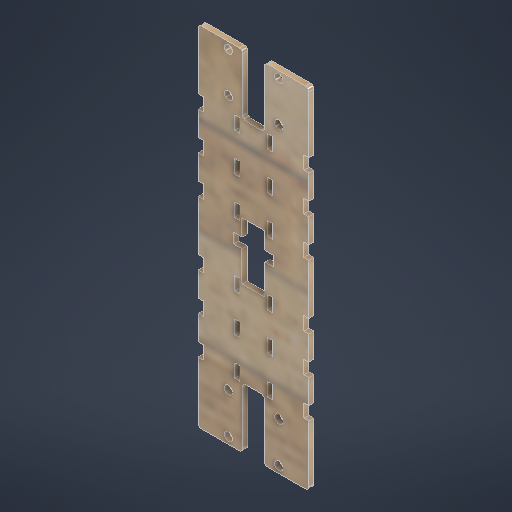
# Autodesk Inventor part: frame_v2
Saved by Autodesk Inventor 2025.3 (Build 293356030, 356C)
## iProperties
Created: 2025-09-03
Part Number: frame_v2
Material: 木材 (楓木)
Document SubType Name: Modeling
Designer: 陳泓任
Density: 0.67 g/cm^3
Appearance: 天然楓木 - 深色亮面處理
Author: 陳泓任
Autodesk Inventor part; units mm, degrees
ref_plane "YZ Plane" through (0, 0, 0) normal (1, 0, 0) x (0, 1, 0)
ref_plane "XZ Plane" through (0, 0, 0) normal (0, 1, 0) x (-1, 0, 0)
ref_plane "XY Plane" through (0, 0, 0) normal (0, 0, 1) x (1, 0, 0)
sketch "草圖1" plane through (0, 0, 0) normal (0, 0, 1) x (1, 0, 0)
  line L0 (-33, -104) -> (33, 104) construction
  line L1 (33, -104) -> (-33, 104) construction
  line L2 (0, 128.5379) -> (0, -160.5456)
  circle A0 centre (-15, 100) radius 2.5
  circle A1 centre (15, 100) radius 2.5
  circle A2 centre (15, 76) radius 2.5
  circle A3 centre (-15, 76) radius 2.5
  line L3 (-33, 68) -> (-30, 68)
  line L4 (-30, 68) -> (-30, 60)
  line L5 (-30, 60) -> (-33, 60)
  line L6 (-33, 102) -> (-33, 68)
  line L7 (-11.2, 68) -> (-8.2, 68)
  line L8 (-8.2, 68) -> (-8.2, 60)
  line L9 (-8.2, 60) -> (-11.2, 60)
  line L10 (-11.2, 60) -> (-11.2, 68)
  line L11 (33, 68) -> (30, 68)
  line L12 (30, 68) -> (30, 60)
  line L13 (30, 60) -> (33, 60)
  line L14 (11.2, 68) -> (8.2, 68)
  line L15 (8.2, 68) -> (8.2, 60)
  line L16 (8.2, 60) -> (11.2, 60)
  line L17 (11.2, 60) -> (11.2, 68)
  line L18 (33, 68) -> (33, 102)
  line L19 (8.2, 45.5) -> (8.2, 37.5)
  line L20 (8.2, 37.5) -> (11.2, 37.5)
  line L21 (11.2, 45.5) -> (8.2, 45.5)
  line L22 (11.2, 37.5) -> (11.2, 45.5)
  line L23 (30, 45.5) -> (30, 37.5)
  line L24 (30, 37.5) -> (33, 37.5)
  line L25 (33, 45.5) -> (30, 45.5)
  line L26 (-8.2, 45.5) -> (-8.2, 37.5)
  line L27 (-8.2, 37.5) -> (-11.2, 37.5)
  line L28 (-11.2, 45.5) -> (-8.2, 45.5)
  line L29 (-11.2, 37.5) -> (-11.2, 45.5)
  line L30 (-30, 45.5) -> (-30, 37.5)
  line L31 (-33, 45.5) -> (-30, 45.5)
  line L32 (-30, 37.5) -> (-33, 37.5)
  line L33 (8.2, 23) -> (8.2, 15)
  line L34 (8.2, 15) -> (11.2, 15)
  line L35 (11.2, 23) -> (8.2, 23)
  line L36 (11.2, 15) -> (11.2, 23)
  line L37 (30, 23) -> (30, 15)
  line L38 (30, 15) -> (33, 15)
  line L39 (33, 23) -> (30, 23)
  line L40 (-8.2, 23) -> (-8.2, 15)
  line L41 (-8.2, 15) -> (-11.2, 15)
  line L42 (-11.2, 23) -> (-8.2, 23)
  line L43 (-11.2, 15) -> (-11.2, 23)
  line L44 (-30, 23) -> (-30, 15)
  line L45 (-33, 23) -> (-30, 23)
  line L46 (-30, 15) -> (-33, 15)
  line L47 (-33, 60) -> (-33, 45.5)
  line L48 (-33, 37.5) -> (-33, 23)
  line L49 (33, 23) -> (33, 37.5)
  line L50 (33, 45.5) -> (33, 60)
  line L51 (-4.5, 68) -> (4.5, 68)
  line L52 (6.5, 70) -> (6.5, 102)
  line L53 (-6.5, 102) -> (-6.5, 70)
  line L54 (-6.5, 68) -> (6.5, 104) construction
  line L55 (6.5, 68) -> (-6.5, 104) construction
  line L56 (31, 104) -> (8.5, 104)
  line L57 (-8.5, 104) -> (-31, 104)
  arc A4 (-6.5, 102) -> (-8.5, 104) centre (-8.5, 102) ccw
  arc A5 (8.5, 104) -> (6.5, 102) centre (8.5, 102) ccw
  arc A6 (-6.5, 70) -> (-4.5, 68) centre (-4.5, 70) ccw
  arc A7 (4.5, 68) -> (6.5, 70) centre (4.5, 70) ccw
  arc A8 (-31, 104) -> (-33, 102) centre (-31, 102) ccw
  arc A9 (33, 102) -> (31, 104) centre (31, 102) ccw
  line L58 (-83.0249, 0) -> (86.2934, 0)
  circle A10 centre (-15, -100) radius 2.5
  circle A11 centre (15, -100) radius 2.5
  circle A12 centre (15, -76) radius 2.5
  circle A13 centre (-15, -76) radius 2.5
  line L59 (-33, -68) -> (-30, -68)
  line L60 (-30, -68) -> (-30, -60)
  line L61 (-30, -60) -> (-33, -60)
  line L62 (-33, -102) -> (-33, -68)
  line L63 (-11.2, -68) -> (-8.2, -68)
  line L64 (-8.2, -68) -> (-8.2, -60)
  line L65 (-8.2, -60) -> (-11.2, -60)
  line L66 (-11.2, -60) -> (-11.2, -68)
  line L67 (33, -68) -> (30, -68)
  line L68 (30, -68) -> (30, -60)
  line L69 (30, -60) -> (33, -60)
  line L70 (8.2, -60) -> (11.2, -60)
  line L71 (11.2, -60) -> (11.2, -68)
  line L72 (8.2, -68) -> (8.2, -60)
  line L73 (11.2, -68) -> (8.2, -68)
  line L74 (33, -68) -> (33, -102)
  line L75 (8.2, -45.5) -> (8.2, -37.5)
  line L76 (8.2, -37.5) -> (11.2, -37.5)
  line L77 (11.2, -45.5) -> (8.2, -45.5)
  line L78 (11.2, -37.5) -> (11.2, -45.5)
  line L79 (30, -45.5) -> (30, -37.5)
  line L80 (30, -37.5) -> (33, -37.5)
  line L81 (33, -45.5) -> (30, -45.5)
  line L82 (-8.2, -45.5) -> (-8.2, -37.5)
  line L83 (-8.2, -37.5) -> (-11.2, -37.5)
  line L84 (-11.2, -45.5) -> (-8.2, -45.5)
  line L85 (-11.2, -37.5) -> (-11.2, -45.5)
  line L86 (-30, -45.5) -> (-30, -37.5)
  line L87 (-33, -45.5) -> (-30, -45.5)
  line L88 (-30, -37.5) -> (-33, -37.5)
  line L89 (8.2, -23) -> (8.2, -15)
  line L90 (8.2, -15) -> (11.2, -15)
  line L91 (11.2, -23) -> (8.2, -23)
  line L92 (11.2, -15) -> (11.2, -23)
  line L93 (30, -23) -> (30, -15)
  line L94 (30, -15) -> (33, -15)
  line L95 (33, -23) -> (30, -23)
  line L96 (-8.2, -23) -> (-8.2, -15)
  line L97 (-8.2, -15) -> (-11.2, -15)
  line L98 (-11.2, -23) -> (-8.2, -23)
  line L99 (-11.2, -15) -> (-11.2, -23)
  line L100 (-30, -23) -> (-30, -15)
  line L101 (-33, -23) -> (-30, -23)
  line L102 (-30, -15) -> (-33, -15)
  line L103 (-33, -60) -> (-33, -45.5)
  line L104 (-33, -37.5) -> (-33, -23)
  line L105 (33, -23) -> (33, -37.5)
  line L106 (33, -45.5) -> (33, -60)
  line L107 (-4.5, -68) -> (4.5, -68)
  line L108 (6.5, -70) -> (6.5, -102)
  line L109 (-6.5, -102) -> (-6.5, -70)
  line L110 (-6.5, -68) -> (6.5, -104) construction
  line L111 (6.5, -68) -> (-6.5, -104) construction
  line L112 (31, -104) -> (8.5, -104)
  line L113 (-8.5, -104) -> (-31, -104)
  arc A14 (-8.5, -104) -> (-6.5, -102) centre (-8.5, -102) ccw
  arc A15 (6.5, -102) -> (8.5, -104) centre (8.5, -102) ccw
  arc A16 (-4.5, -68) -> (-6.5, -70) centre (-4.5, -70) ccw
  arc A17 (6.5, -70) -> (4.5, -68) centre (4.5, -70) ccw
  arc A18 (-33, -102) -> (-31, -104) centre (-31, -102) ccw
  arc A19 (31, -104) -> (33, -102) centre (31, -102) ccw
  line L114 (-31, -104) -> (-8.5, -104)
  line L115 (8.5, -104) -> (31, -104)
  line L116 (-6.85, -17.1) -> (6.85, -17.1)
  line L117 (6.85, 17.1) -> (-6.85, 17.1)
  line L118 (-6.85, -17.1) -> (6.85, 17.1) construction
  line L119 (6.85, -17.1) -> (-6.85, 17.1) construction
  line L120 (11.85, 1.05) -> (11.85, 7.05)
  line L121 (-11.85, 7.05) -> (-11.85, 1.05)
  line L122 (-11.85, 1.05) -> (11.85, 7.05) construction
  line L123 (11.85, 1.05) -> (-11.85, 7.05) construction
  line L124 (-6.85, 17.1) -> (-6.85, 7.05)
  line L125 (-6.85, 1.05) -> (-6.85, -17.1)
  line L126 (6.85, -17.1) -> (6.85, 1.05)
  line L127 (6.85, 7.05) -> (6.85, 17.1)
  line L128 (11.85, 7.05) -> (6.85, 7.05)
  line L129 (6.85, 1.05) -> (11.85, 1.05)
  line L130 (-11.85, 1.05) -> (-6.85, 1.05)
  line L131 (-6.85, 7.05) -> (-11.85, 7.05)
  line L132 (-33, 15) -> (-33, -15)
  line L133 (-33, -23) -> (-33, -37.5)
  line L134 (-33, -45.5) -> (-33, -60)
  line L135 (-33, -68) -> (-33, -102)
  line L136 (33, -102) -> (33, -68)
  line L137 (33, -60) -> (33, -45.5)
  line L138 (33, -37.5) -> (33, -23)
  line L139 (33, -15) -> (33, 15)
  line L140 (-65.8128, 14.982) -> (72.6132, 14.982) construction
  point P0 (0, 0)
  point P1 (0, 86.5078)
  point P2 (0, 86)
  point P3 (0, -86.5078)
  point P4 (0, -86)
  point P5 (0, 4.05)
  point P6 (11.85, 4.05)
  dimension "d0" = 66
  dimension "d1" = 208
  dimension "d6" = 5
  dimension "d8" = 30
  dimension "d9" = 24
  dimension "d10" = 3
  dimension "d11" = 8
  dimension "d12" = 8
  dimension "d13" = 3
  dimension "d14" = 18.8
  dimension "d17" = 22.5
  dimension "d22" = 13
  dimension "d23" = 4
  dimension "d24" = 2
  dimension "d25" = 2
  dimension "d26" = 34.2
  dimension "d27" = 13.7
  dimension "d28" = 6
  dimension "d30" = 23.7
  dimension "d31" = 10.05
  dimension "d37" = 2.118
  dimension "d38" = -0.018
  constraints: 282 end point, 84 symmetric about line, 67 parallel, 29 point on line, 24 point on circle, 21 perpendicular, 20 centre point, 12 tangent, 10 horizontal, 9 midpoint, 7 equal radius, 5 collinear, 2 vertical, 1 vertical alignment, 72 other
  measures "d0" distance of L0.end L1.end
  measures "d1" distance of L1.start L0.end
  measures "d6" diameter of A0
  measures "d8" distance of A2.centre A3.centre
  measures "d9" distance of A1.centre A2.centre
  measures "d10" distance of L4.end L5.end
  measures "d11" distance of L3.end L4.end
  measures "d12" distance from line of L3 A3.centre
  measures "d13" distance of L7.start L7.end
  measures "d14" distance between parallel lines of L4 L10
  measures "d17" distance of L16.start L19.end
  measures "d22" distance of L54.start L55.start
  measures "d23" distance from line of A0.centre L57
  measures "d24" radius of A4
  measures "d25" radius of A8
  measures "d26" distance of L116.end L117.start
  measures "d27" distance of L117.start L117.end
  measures "d28" distance of L120.start L120.end
  measures "d30" distance from line of point (11.85, 4.05) L121
  measures "d31" distance between parallel lines of L131 L117
  measures "d37" distance between parallel lines of L140 L117
  measures "d38" distance between parallel lines of L34 L140
extrude "擠出1" add sketch "草圖1" along normal blind 3 contours L51 A7 L52 A5 L56 A9 L18 L11 L12 L13 L50 L25 L23 L24 L49 L39 L37 L38 L139 L58 L126 L129 L120 L128 L127 L117 L2 | L2 L117 L124 L131 L121 L130 L125 L58 L132 L46 L44 L45 L48 L32 L30 L31 L47 L5 L4 L3 L6 A8 L57 A4 L53 A6 L51 | L116 L126 L58 L139 L94 L93 L95 L105 L80 L79 L81 L106 L69 L68 L67 L74 A19 L112 A15 L108 A17 L107 L2 | L2 L107 A16 L109 A14 L113 A18 L62 L59 L60 L61 L103 L87 L86 L88 L104 L101 L100 L102 L132 L58 L125 L116
sketch "草圖3" plane through (0, 0, 3) normal (0, 0, 1) x (1, 0, 0)
  line L0 (-88.1264, 0) -> (75.7938, 0)
  line L1 (0, 123.8394) -> (0, -129.4918)
  point P0 (0, 0)
  constraints: 4 end point, 2 point on line, 1 horizontal, 1 perpendicular
